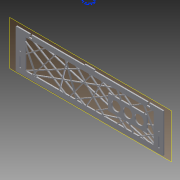
# Autodesk Inventor part: Panel_back
Saved by Autodesk Inventor 2013 (Build 170138000, 138)
## iProperties
Created: 2013-02-02
Part Number: Panel_back
Material: Aluminum 6061
Document SubType Name: Modeling
Designer: xylzlyx
Density: 1 g/cm^3
Author: xylzlyx
Autodesk Inventor part; units mm, degrees
ref_plane "YZ Plane" through (0, 0, 0) normal (1, 0, 0) x (0, 1, 0)
ref_plane "XZ Plane" through (0, 0, 0) normal (0, 1, 0) x (-1, 0, 0)
ref_plane "XY Plane" through (0, 0, 0) normal (0, 0, 1) x (1, 0, 0)
ref_plane "Work Plane1" through (-16.0071, 0, -12.7) normal (0, 0, 1) x (1, 0, 0)
sketch "Sketch1" plane through (-16.0071, 0, -12.7) normal (0, 0, 1) x (1, 0, 0)
  line L0 (0, -104.216) -> (0, -100.9921) construction
  line L1 (0, -100.9921) -> (381, -100.9921) construction
  line L2 (381, -100.9921) -> (381, -104.216) construction
  line L3 (381, -104.216) -> (0, -104.216) construction
  line L4 (381, 3.175) -> (381, 0) construction
  line L5 (381, 0) -> (0, 0) construction
  line L6 (0, 0) -> (0, 3.175) construction
  line L7 (0, 3.175) -> (381, 3.175) construction
  line L8 (381, -100.9921) -> (0, -100.9921)
  line L9 (0, -100.9921) -> (0, 0)
  line L10 (0, 0) -> (381, 0)
  line L11 (381, 0) -> (381, -100.9921)
  constraints: 24 end point, 5 horizontal, 4 coincident, 4 vertical, 2 parallel, 1 perpendicular, 7 other
extrude "BackPanel" add sketch "Sketch1" along normal blind 3.175
fillet "CornerFillet" radius 1 4 edges at (364.9929, -100.9921, -11.1125) (364.9929, 0, -11.1125) (-16.0071, 0, -11.1125) (-16.0071, -100.9921, -11.1125)
sketch "ScrewSlotSketch" plane through (-16.0071, 0, -9.525) normal (0, 0, 1) x (1, 0, 0)
  line L0 (0, -104.7759) -> (0, -101.5519) construction
  line L1 (0, -101.5519) -> (381, -101.5519) construction
  line L2 (381, -101.5519) -> (381, -104.7759) construction
  line L3 (381, -104.7759) -> (0, -104.7759) construction
  line L4 (381, 0) -> (0, 0) construction
  line L5 (0, 0) -> (0, 3.175) construction
  line L6 (0, 3.175) -> (381, 3.175) construction
  line L7 (381, 3.175) -> (381, 0) construction
  line L8 (341.0013, 3.175) -> (341.0013, -8.89)
  line L9 (341.0013, 3.175) -> (344.7986, 3.175)
  line L10 (344.7986, 3.175) -> (344.7986, -8.89)
  line L11 (344.7986, -8.89) -> (341.0013, -8.89)
  line L12 (342.9, -8.89) -> (342.9, 3.175) construction
  line L13 (346.9957, -8.89) -> (338.8042, -8.89)
  line L14 (338.8042, -8.89) -> (338.8042, -5.8579)
  line L15 (338.8042, -5.8579) -> (346.9957, -5.8579)
  line L16 (346.9957, -5.8579) -> (346.9957, -8.89)
  line L17 (36.2014, -8.89) -> (36.2014, 3.175)
  line L18 (36.2014, 3.175) -> (39.9987, 3.175)
  line L19 (39.9987, 3.175) -> (39.9987, -8.89)
  line L20 (39.9987, -8.89) -> (36.2014, -8.89)
  line L21 (42.1958, -8.89) -> (34.0043, -8.89)
  line L22 (42.1958, -8.89) -> (42.1958, -5.8579)
  line L23 (42.1958, -5.8579) -> (34.0043, -5.8579)
  line L24 (34.0043, -5.8579) -> (34.0043, -8.89)
  line L25 (368.3, -48.0974) -> (368.3, -1) projected
  line L26 (12.7, -1) -> (12.7, -48.0974) projected
  line L27 (368.3, -48.0974) -> (368.3, -1) projected
  point P0 (16.0071, 0)
  point P1 (38.1, 3.175)
  point P2 (38.1, -8.89)
  dimension "d3" = 12.065
  dimension "d5" = 3.7973
  dimension "d7" = 8.1915
  dimension "d8" = 3.0321
  dimension "d9" = 12.065
  dimension "d10" = 3.7973
  dimension "d12" = 8.1915
  dimension "d13" = 3.0321
  dimension "d22" = 25.4
  dimension "d23" = 25.4
  constraints: 50 end point, 13 parallel, 6 midpoint, 4 horizontal, 4 vertical, 3 collinear, 2 point on line, 1 perpendicular, 8 other
  measures "d3" distance of L8.start L8.end
  measures "d5" distance of L8.start L9.end
  measures "d7" distance of L13.start L13.end
  measures "d8" distance of L15.end L13.start
  measures "d9" distance of L17.start L17.end
  measures "d10" distance of L17.end L18.end
  measures "d12" distance of L21.start L21.end
  measures "d13" distance of L21.start L22.end
  measures "d22" distance between parallel lines of L12 L25
  measures "d23" distance from line of L26 point (38.1, 3.175)
extrude "ScrewSlotExtrusion" cut sketch "ScrewSlotSketch" against normal blind 3.175
fillet "SlotFillets" radius 0.5 16 edges at (328.7916, -5.8579, -11.1125) (328.7916, 0, -11.1125) (324.9943, 0, -11.1125) (324.9943, -5.8579, -11.1125) (330.9887, -5.8579, -11.1125) (322.7972, -5.8579, -11.1125) (330.9887, -8.89, -11.1125) (322.7972, -8.89, -11.1125) (20.1943, -5.8579, -11.1125) (17.9972, -5.8579, -11.1125) (20.1943, 0, -11.1125) (17.9972, -8.89, -11.1125) (23.9916, -5.8579, -11.1125) (23.9916, 0, -11.1125) (26.1887, -8.89, -11.1125) (26.1887, -5.8579, -11.1125)
sketch "ScrewHoleSketch" plane through (-16.0071, 0, -9.525) normal (0, 0, 1) x (1, 0, 0)
  line L0 (368.3, -48.5974) -> (371.475, -48.5974) projected
  line L1 (371.475, -52.3947) -> (368.3, -52.3947) projected
  line L2 (12.7, -52.3947) -> (9.525, -52.3947) projected
  line L3 (9.525, -48.5974) -> (12.7, -48.5974) projected
  line L4 (368.3, -48.5974) -> (368.3, -52.3947) construction
  line L5 (12.7, -48.5974) -> (12.7, -52.3947) construction
  line L6 (36.2014, -5.3579) -> (36.2014, -0.5) projected
  line L7 (344.7986, -0.5) -> (344.7986, -5.3579) projected
  point P0 (16.0071, 0)
  point P1 (369.8875, -50.496)
  point P2 (11.1125, -50.496)
  point P3 (368.3, -50.496)
  point P4 (369.8875, -48.5974)
  point P5 (11.1125, -48.5974)
  point P6 (12.7, -50.496)
  constraints: 4 end point, 4 midpoint, 3 parallel, 2 horizontal alignment, 2 vertical alignment
hole "Hole1" at (353.8804, -50.496, -9.525) at (-4.8946, -50.496, -9.525) direction (0, 0, -1) diameter 3.7973 end through all
sketch "BottomTabSketch" plane through (24.4916, 0, -12.7) normal (0, 1, 0) x (1, 0, 0)
  line L0 (137.3013, -3.175) -> (162.7013, -3.175)
  line L1 (162.7013, -3.175) -> (162.7013, 0)
  line L2 (162.7013, 0) -> (137.3013, 0)
  line L3 (137.3013, 0) -> (137.3013, -3.175)
  line L4 (137.5473, -3.429) -> (162.4553, -3.429) projected
  line L5 (137.0473, -0.246) -> (137.0473, -2.929) projected
  point P0 (0, 0)
  point P1 (-24.4916, -12.7)
  point P2 (150.0013, -3.175)
  point P3 (150.0013, -3.429)
  point P4 (137.3013, -1.5875)
  point P5 (137.0473, -1.5875)
  dimension "d32" = 25.4
  constraints: 8 end point, 4 midpoint, 2 horizontal alignment, 2 parallel, 1 horizontal, 1 perpendicular, 1 vertical alignment
  measures "d32" distance of L1.end L2.end
extrude "BottomTab" add sketch "BottomTabSketch" along normal blind 3.175
fillet "BottomTabFillet" radius 0.5 4 edges at (161.7929, 0, -11.1125) (161.7929, 3.175, -11.1125) (187.1929, 0, -11.1125) (187.1929, 3.175, -11.1125)
sketch "SlotSketch" plane through (-16.0071, 0, -9.525) normal (0, 0, 1) x (1, 0, 0)
  circle A0 centre (369.8875, -50.496) radius 1.8986 projected
  circle A1 centre (11.1125, -50.496) radius 1.8986 projected
  line L0 (0, -104.7759) -> (0, -101.5519) construction
  line L1 (0, -101.5519) -> (381, -101.5519) construction
  line L2 (381, -101.5519) -> (381, -104.7759) construction
  line L3 (381, -104.7759) -> (0, -104.7759) construction
  line L4 (371.729, -88.6981) -> (368.046, -88.6981)
  line L5 (368.046, -88.6981) -> (368.046, -62.7901)
  line L6 (368.046, -62.7901) -> (371.729, -62.7901)
  line L7 (371.729, -62.7901) -> (371.729, -88.6981)
  line L8 (12.954, -88.6981) -> (9.271, -88.6981)
  line L9 (9.271, -88.6981) -> (9.271, -62.7901)
  line L10 (9.271, -62.7901) -> (12.954, -62.7901)
  line L11 (12.954, -62.7901) -> (12.954, -88.6981)
  line L12 (1, -100.9921) -> (380, -100.9921) projected
  line L13 (203.2, 0.5) -> (203.2, 2.675) projected
  line L14 (11.1125, -50.496) -> (11.1125, -100.9921) construction
  line L15 (369.8875, -50.496) -> (369.8875, -100.9921) construction
  point P0 (16.0071, 0)
  point P1 (11.1125, -75.7441)
  point P2 (12.954, -75.7441)
  point P3 (11.1125, -62.7901)
  point P4 (369.8875, -75.7441)
  point P5 (371.729, -75.7441)
  point P6 (369.8875, -62.7901)
  dimension "d37" = 25.908
  dimension "d39" = 3.683
  dimension "d40" = 25.908
  dimension "d41" = 3.683
  constraints: 28 end point, 6 midpoint, 6 parallel, 4 horizontal, 2 horizontal alignment, 2 perpendicular, 2 point on line, 2 vertical, 2 vertical alignment, 4 other
  measures "d37" distance of L4.end L5.end
  measures "d39" distance of L4.start L4.end
  measures "d40" distance of L10.end L8.start
  measures "d41" distance of L8.start L8.end
extrude "Slots" cut sketch "SlotSketch" against normal blind 3.175 contours L4 L5 L6 L7 | L8 L9 L10 L11
fillet "Fillet4" radius 0.5 8 edges at (355.7219, -88.6981, -11.1125) (352.0389, -88.6981, -11.1125) (352.0389, -62.7901, -11.1125) (355.7219, -62.7901, -11.1125) (-6.7361, -62.7901, -11.1125) (-3.0531, -62.7901, -11.1125) (-6.7361, -88.6981, -11.1125) (-3.0531, -88.6981, -11.1125)
sketch "Sketch6" plane through (-16.0071, 0, -9.525) normal (0, 0, 1) x (1, 0, 0)
  line L0 (1, -100.9921) -> (380, -100.9921) projected
  line L1 (380, 0) -> (345.2986, 0) projected
  circle A0 centre (369.8875, -50.496) radius 1.8986 projected
  circle A1 centre (11.1125, -50.496) radius 1.8986 projected
  line L2 (357.1875, -88.2921) -> (23.8125, -88.2921)
  line L3 (23.8125, -88.2921) -> (23.8125, -12.7)
  line L4 (23.8125, -12.7) -> (357.1875, -12.7)
  line L5 (357.1875, -12.7) -> (357.1875, -88.2921)
  point P0 (16.0071, 0)
  dimension "d45" = 12.7
  dimension "d46" = 12.7
  dimension "d47" = 12.7
  dimension "d48" = 12.7
  constraints: 8 end point, 2 parallel, 1 horizontal, 1 perpendicular
  measures "d45" distance from line of L0 L2.start
  measures "d46" distance from line of L1 L4.end
  measures "d47" distance from line of A0.centre L5
  measures "d48" horizontal distance of A1.centre L3.end
extrude "InsideGap" cut sketch "Sketch6" against normal blind 25.4 contours L2 L3 L4 L5
fillet "InsideGapFillet" radius 0.5 4 edges at (341.1804, -88.2921, -11.1125) (341.1804, -12.7, -11.1125) (7.8054, -12.7, -11.1125) (7.8054, -88.2921, -11.1125)
sketch "Sketch7" plane through (-16.0071, 0, -9.525) normal (0, 0, 1) x (1, 0, 0)
  line L0 (357.1875, -13.2) -> (357.1875, -87.7921) projected
  line L1 (356.6875, -88.2921) -> (24.3125, -88.2921) projected
  line L2 (23.8125, -87.7921) -> (23.8125, -13.2) projected
  line L3 (24.3125, -12.7) -> (356.6875, -12.7) projected
  line L4 (340.5013, 0) -> (203.7, 0) projected
  line L5 (354.4479, -12.7) -> (264.3608, -88.2921)
  line L6 (327.4775, -12.7) -> (206.5049, -88.2921)
  line L7 (285.5675, -12.7) -> (154.6382, -88.2921)
  line L8 (254.9043, -12.7) -> (47.2168, -88.2921)
  line L9 (225.9343, -12.7) -> (182.8154, -88.2921)
  line L10 (169.3262, -12.7) -> (27.1582, -88.2921)
  line L11 (132.4925, -12.7) -> (113.0758, -88.2921)
  line L12 (77.2875, -12.7) -> (23.8125, -52.9963)
  line L13 (357.1875, -66.5903) -> (320.5833, -88.2921)
  line L14 (357.1875, -66.5903) -> (357.1875, -64.228)
  line L15 (357.1875, -64.228) -> (316.5989, -88.2921)
  line L16 (316.5989, -88.2921) -> (320.5833, -88.2921)
  line L17 (351.2867, -12.7) -> (261.1996, -88.2921)
  line L18 (261.1996, -88.2921) -> (264.3608, -88.2921)
  line L19 (354.4479, -12.7) -> (351.2867, -12.7)
  line L20 (327.4775, -12.7) -> (323.643, -12.7)
  line L21 (323.643, -12.7) -> (202.6704, -88.2921)
  line L22 (202.6704, -88.2921) -> (206.5049, -88.2921)
  line L23 (285.5675, -12.7) -> (281.5035, -12.7)
  line L24 (281.5035, -12.7) -> (150.5742, -88.2921)
  line L25 (150.5742, -88.2921) -> (154.6382, -88.2921)
  line L26 (254.9043, -12.7) -> (248.9631, -12.7)
  line L27 (248.9631, -12.7) -> (41.2756, -88.2921)
  line L28 (41.2756, -88.2921) -> (47.2168, -88.2921)
  line L29 (225.9343, -12.7) -> (223.595, -12.7)
  line L30 (223.595, -12.7) -> (180.476, -88.2921)
  line L31 (180.476, -88.2921) -> (182.8154, -88.2921)
  line L32 (169.3262, -12.7) -> (164.998, -12.7)
  line L33 (164.998, -12.7) -> (22.83, -88.2921)
  line L34 (22.83, -88.2921) -> (27.1582, -88.2921)
  line L35 (132.4925, -12.7) -> (130.3945, -12.7)
  line L36 (130.3945, -12.7) -> (110.9779, -88.2921)
  line L37 (110.9779, -88.2921) -> (113.0758, -88.2921)
  line L38 (77.2875, -12.7) -> (73.911, -12.7)
  line L39 (73.911, -12.7) -> (23.8125, -50.452)
  line L40 (23.8125, -50.452) -> (23.8125, -52.9963)
  line L41 (195.7846, -12.7) -> (140.0963, -88.2921)
  line L42 (140.0963, -88.2921) -> (137.5725, -88.2921)
  line L43 (137.5725, -88.2921) -> (193.2608, -12.7)
  line L44 (193.2608, -12.7) -> (195.7846, -12.7)
  line L45 (103.9917, -12.7) -> (43.8325, -88.2921)
  line L46 (43.8325, -88.2921) -> (41.2356, -88.2921)
  line L47 (41.2356, -88.2921) -> (101.3947, -12.7)
  line L48 (101.3947, -12.7) -> (103.9917, -12.7)
  arc A0 (357.1875, -13.2) -> (356.6875, -12.7) centre (356.6875, -13.2) ccw projected
  line L49 (357.1875, -46.5241) -> (225.1649, -88.2921)
  line L50 (357.1875, -46.5241) -> (357.1875, -44.3928)
  line L51 (357.1875, -44.3928) -> (218.4282, -88.2921)
  line L52 (218.4282, -88.2921) -> (225.1649, -88.2921)
  point P0 (16.0071, 0)
  dimension "d52" = 2.2396
  dimension "d53" = 29.21
  dimension "d54" = 71.12
  dimension "d55" = 101.7832
  dimension "d56" = 130.7532
  dimension "d57" = 187.3613
  dimension "d58" = 224.195
  dimension "d59" = 279.4
  dimension "d60" = 53.3903
  dimension "d61" = 59.337
  dimension "d62" = 140
  dimension "d63" = 148
  dimension "d64" = 150
  dimension "d65" = 160
  dimension "d66" = 119.701
  dimension "d67" = 152
  dimension "d68" = 104.406
  dimension "d69" = 143
  dimension "d70" = 2.032
  dimension "d71" = 2.032
  dimension "d72" = 2.032
  dimension "d73" = 2.032
  dimension "d74" = 2.032
  dimension "d75" = 2.032
  dimension "d76" = 2.032
  dimension "d77" = 2.032
  dimension "d78" = 2.032
  dimension "d79" = 2.032
  dimension "d80" = 160.9029
  dimension "d81" = 126.379
  dimension "d82" = 252.6958
  dimension "d83" = 128.514
  dimension "d84" = 2.032
  dimension "d122" = 33.324
  dimension "d123" = 72.444
  dimension "d124" = 2.032
  constraints: 96 end point, 17 parallel, 14 horizontal, 3 collinear, 3 point on line, 27 other
  measures "d52" distance of L5.start A0.end
  measures "d53" distance of L6.start A0.end
  measures "d54" distance of L7.start A0.end
  measures "d55" distance of L8.start A0.end
  measures "d56" distance of L9.start A0.end
  measures "d57" distance of L10.start A0.end
  measures "d58" distance of L11.start A0.end
  measures "d59" distance of L12.start A0.end
  measures "d60" distance of L0.start L13.start
  measures "d61" angle of L0 L13
  measures "d62" angle to the sketch x axis of L5
  measures "d63" angle to the sketch x axis of L6
  measures "d64" angle to the sketch x axis of L7
  measures "d65" angle to the sketch x axis of L8
  measures "d66" angle to the sketch x axis of L9
  measures "d67" angle to the sketch x axis of L10
  measures "d68" angle to the sketch x axis of L11
  measures "d69" angle to the sketch x axis of L12
  measures "d70" distance between parallel lines of L15 L13
  measures "d71" distance between parallel lines of L5 L17
  measures "d72" distance between parallel lines of L6 L21
  measures "d73" distance between parallel lines of L7 L24
  measures "d74" distance between parallel lines of L8 L27
  measures "d75" distance between parallel lines of L9 L30
  measures "d76" distance between parallel lines of L10 L33
  measures "d77" distance between parallel lines of L11 L36
  measures "d78" distance between parallel lines of L12 L39
  measures "d79" distance between parallel lines of L41 L43
  measures "d80" distance of A0.end L41.start
  measures "d81" angle to the sketch x axis of L41
  measures "d82" distance of A0.end L45.start
  measures "d83" angle to the sketch x axis of L45
  measures "d84" distance between parallel lines of L45 L47
  measures "d122" vertical distance of A0.centre L49.start
  measures "d123" angle of L0 L49
  measures "d124" distance between parallel lines of L49 L51
extrude "Hash1" add sketch "Sketch7" against normal blind 3.175 contours L0 L49 L5 L51 | L51 L17 L3 L5 | L5 L49 L17 L51 | L0 L13 L1 L15 | L5 L1 L17 L49 | L17 L49 L1 L51 | L6 L1 L21 L3 | L7 L9 L24 L3 | L1 L30 L7 L9 | L7 L30 L24 L9 | L8 L9 L27 L3 | L24 L30 L8 L9 | L7 L1 L24 L30 | L8 L30 L27 L9 | L9 L27 L30 L3 | L8 L41 L27 L30 | L1 L43 L8 L41 | L8 L43 L27 L41 | L41 L27 L43 L3 | L8 L11 L27 L43 | L1 L36 L8 L11 | L8 L36 L27 L11 | L10 L11 L33 L3 | L27 L36 L10 L11 | L8 L1 L45 L27 L36 | L10 L36 L33 L11 | L1 L27 L45 | L11 L33 L36 L3 | L10 L45 L33 L36 | L27 L1 L47 L10 L45 | L10 L47 L33 L45 | L45 L33 L47 L3 | L10 L1 L34 L33 L47 | L12 L2 L39 L3
sketch "Sketch8" plane through (-16.0071, 0, -9.525) normal (0, 0, 1) x (1, 0, 0)
  line L0 (77.2875, -12.7) -> (101.3947, -12.7) projected
  line L1 (169.3262, -12.7) -> (193.2608, -12.7) projected
  line L2 (137.5725, -88.2921) -> (113.0758, -88.2921) projected
  line L3 (110.9779, -88.2921) -> (320.5833, -88.2921) projected
  line L4 (356.6875, -88.2921) -> (140.0963, -88.2921) projected
  line L5 (357.1875, -66.5903) -> (357.1875, -87.7921) projected
  line L6 (316.5989, -88.2921) -> (206.5049, -88.2921) projected
  line L7 (261.1996, -88.2921) -> (154.6382, -88.2921) projected
  line L8 (285.5675, -12.7) -> (323.643, -12.7) projected
  line L9 (254.9043, -12.7) -> (281.5035, -12.7) projected
  line L10 (150.5742, -88.2921) -> (182.8154, -88.2921) projected
  line L11 (132.4925, -12.7) -> (164.998, -12.7) projected
  line L12 (225.9343, -12.7) -> (248.9631, -12.7) projected
  line L13 (23.8125, -50.452) -> (23.8125, -13.2) projected
  line L14 (24.3125, -12.7) -> (73.911, -12.7) projected
  line L15 (327.4775, -12.7) -> (351.2867, -12.7) projected
  line L16 (340.5013, 0) -> (203.7, 0) projected
  line L17 (23.8125, -34.0474) -> (50.1687, -88.2921)
  line L18 (23.8125, -24.8637) -> (123.9909, -88.2921)
  line L19 (42.1433, -12.7) -> (173.0726, -88.2921)
  line L20 (76.4841, -12.7) -> (332.9933, -88.2921)
  line L21 (126.5475, -12.7) -> (155.5646, -88.2921)
  line L22 (153.8525, -12.7) -> (225.0869, -88.2921)
  line L23 (187.5335, -12.7) -> (281.551, -88.2921)
  line L24 (218.779, -12.7) -> (357.1875, -88.2921)
  line L25 (259.8239, -12.7) -> (300.7816, -88.2921)
  line L26 (273.2325, -12.7) -> (357.1875, -77.3074)
  line L27 (357.1875, -61.6757) -> (328.9114, -12.7)
  line L28 (357.1875, -61.6757) -> (357.1875, -57.6117)
  line L29 (357.1875, -57.6117) -> (331.2577, -12.7)
  line L30 (331.2577, -12.7) -> (328.9114, -12.7)
  line L31 (300.7816, -88.2921) -> (303.0927, -88.2921)
  line L32 (303.0927, -88.2921) -> (262.135, -12.7)
  line L33 (262.135, -12.7) -> (259.8239, -12.7)
  line L34 (281.551, -88.2921) -> (284.7939, -88.2921)
  line L35 (284.7939, -88.2921) -> (190.7764, -12.7)
  line L36 (190.7764, -12.7) -> (187.5335, -12.7)
  line L37 (225.0869, -88.2921) -> (227.8789, -88.2921)
  line L38 (227.8789, -88.2921) -> (156.6446, -12.7)
  line L39 (156.6446, -12.7) -> (153.8525, -12.7)
  line L40 (155.5646, -88.2921) -> (157.7411, -88.2921)
  line L41 (157.7411, -88.2921) -> (128.7241, -12.7)
  line L42 (128.7241, -12.7) -> (126.5475, -12.7)
  line L43 (332.9933, -88.2921) -> (340.1817, -88.2921)
  line L44 (340.1817, -88.2921) -> (83.6725, -12.7)
  line L45 (83.6725, -12.7) -> (76.4841, -12.7)
  line L46 (123.9909, -88.2921) -> (127.7895, -88.2921)
  line L47 (127.7895, -88.2921) -> (23.8125, -22.4586)
  line L48 (23.8125, -22.4586) -> (23.8125, -24.8637)
  line L49 (173.0726, -88.2921) -> (177.1366, -88.2921)
  line L50 (177.1366, -88.2921) -> (46.2073, -12.7)
  line L51 (46.2073, -12.7) -> (42.1433, -12.7)
  line L52 (50.1687, -88.2921) -> (52.4278, -88.2921)
  line L53 (52.4278, -88.2921) -> (23.8125, -29.3978)
  line L54 (23.8125, -29.3978) -> (23.8125, -34.0474)
  line L55 (195.7846, -12.7) -> (223.595, -12.7) projected
  line L56 (357.1875, -77.3074) -> (357.1875, -74.7434)
  line L57 (357.1875, -74.7434) -> (276.5644, -12.7)
  line L58 (276.5644, -12.7) -> (273.2325, -12.7)
  line L59 (357.1875, -88.2921) -> (357.1875, -85.9768)
  line L60 (357.1875, -85.9768) -> (223.0183, -12.7)
  line L61 (223.0183, -12.7) -> (218.779, -12.7)
  point P0 (43.8325, -88.2921)
  point P1 (158.6823, -88.2921)
  point P2 (16.0071, 0)
  dimension "d87" = 20.8474
  dimension "d88" = 11.6637
  dimension "d89" = 154.086
  dimension "d90" = 122.34
  dimension "d91" = 17.8308
  dimension "d92" = 52.1716
  dimension "d93" = 150
  dimension "d94" = 163.58
  dimension "d95" = 102.235
  dimension "d96" = 111
  dimension "d97" = 129.54
  dimension "d98" = 133.3
  dimension "d99" = 163.221
  dimension "d100" = 141.2
  dimension "d101" = 194.4665
  dimension "d103" = 235.5114
  dimension "d104" = 118.45
  dimension "d105" = 248.92
  dimension "d106" = 142.42
  dimension "d107" = 304.5989
  dimension "d108" = 120
  dimension "d109" = 2.032
  dimension "d111" = 2.032
  dimension "d112" = 2.032
  dimension "d114" = 2.032
  dimension "d115" = 2.032
  dimension "d116" = 2.032
  dimension "d117" = 2.032
  dimension "d118" = 2.032
  dimension "d119" = 2.032
  dimension "d125" = 2.032
  dimension "d126" = 2.032
  constraints: 88 end point, 23 point on line, 20 collinear, 13 parallel
  measures "d87" distance of L13.end L17.start
  measures "d88" distance of L13.end L18.start
  measures "d89" angle of L13 L17
  measures "d90" angle of L13 L18
  measures "d91" distance of L14.start L19.start
  measures "d92" distance of L14.start L20.start
  measures "d93" angle of L14 L19
  measures "d94" angle of L0 L20
  measures "d95" distance of L14.start L21.start
  measures "d96" angle of L11 L21
  measures "d97" distance of L14.start L22.start
  measures "d98" angle of L11 L22
  measures "d99" distance of L14.start L23.start
  measures "d100" angle of L1 L23
  measures "d101" distance of L14.start L24.start
  measures "d103" distance of L14.start L25.start
  measures "d104" angle of L12 L25
  measures "d105" distance of L14.start L26.start
  measures "d106" angle of L8 L26
  measures "d107" distance of L14.start L27.end
  measures "d108" angle of L15 L27
  measures "d109" distance between parallel lines of L27 L29
  measures "d111" distance between parallel lines of L25 L32
  measures "d112" distance between parallel lines of L23 L35
  measures "d114" distance between parallel lines of L22 L38
  measures "d115" distance between parallel lines of L21 L41
  measures "d116" distance between parallel lines of L20 L44
  measures "d117" distance between parallel lines of L18 L47
  measures "d118" distance between parallel lines of L19 L50
  measures "d119" distance between parallel lines of L17 L53
  measures "d125" distance between parallel lines of L26 L57
  measures "d126" distance between parallel lines of L24 L60
extrude "Hash2" add sketch "Sketch8" against normal blind 3.175 contours L0 L44 L21 L20 L45 | L44 L41 L20 L21 | L21 L42 L41 L44 | L20 L41 L50 L21 | L44 L22 L20 L41 | L50 L41 L19 L21 | L21 L19 L14 L50 | L44 L38 L20 L22 | L22 L11 L38 L44 | L20 L38 L3 L22 | L50 L3 L19 L41 | L19 L41 L3 L21 | L44 L23 L20 L38 | L44 L35 L20 L23 | L23 L1 L35 L44 | L20 L35 L3 L23 | L44 L25 L20 L35 | L44 L32 L20 L25 | L25 L24 L32 L44 | L20 L32 L3 L25 | L25 L60 L32 L24 | L24 L55 L60 L25 | L44 L4 L20 L32 | L32 L60 L5 L59 L24 | L25 L9 L32 L60 | L9 L57 L5 L26 | L2 L18 L13 L47 | L13 L53 L52 L17 | L15 L29 L28 L27
sketch "Sketch9" plane through (-16.0071, 0, -9.525) normal (0, 0, 1) x (1, 0, 0)
  circle A0 centre (369.8875, -50.496) radius 1.8986 projected
  line L0 (1, -100.9921) -> (380, -100.9921) projected
  line L1 (381, -99.9921) -> (381, -1) projected
  line L2 (380, 0) -> (345.2986, 0) projected
  line L3 (339.0875, -70.496) -> (239.0875, -70.496)
  line L4 (239.0875, -70.496) -> (239.0875, -30.496)
  line L5 (239.0875, -30.496) -> (339.0875, -30.496)
  line L6 (339.0875, -30.496) -> (339.0875, -70.496)
  point P0 (16.0071, 0)
  point P1 (289.0875, -50.496)
  point P2 (259.0875, -50.496)
  point P3 (319.0875, -50.496)
  point P4 (339.0875, -50.496)
  point P5 (289.0875, -70.496)
  dimension "d127" = 30
  dimension "d129" = 30
  dimension "d130" = 50.8
  dimension "d131" = 20
  dimension "d132" = 20
  constraints: 8 end point, 4 horizontal alignment, 4 parallel, 2 midpoint, 1 vertical alignment
  measures "d127" distance of point (289.087, -50.496) point (319.087, -50.496)
  measures "d129" distance of point (289.087, -50.496) point (259.087, -50.496)
  measures "d130" distance of point (319.087, -50.496) A0.centre
  measures "d131" distance from line of L6 point (319.087, -50.496)
  measures "d132" distance from line of L3 point (319.087, -50.496)
extrude "BackButtonMount" add sketch "Sketch9" against normal blind 3.175 contours L3 L4 L5 L6
sketch "Sketch10" plane through (-16.0071, 0, -9.525) normal (0, 0, 1) x (1, 0, 0)
  circle A0 centre (369.8875, -50.496) radius 1.8986 projected
  point P0 (16.0071, 0)
  point P1 (319.0875, -50.496)
  point P2 (289.0875, -50.496)
  point P3 (259.0875, -50.496)
  point P4 (289.0875, -50.496)
  dimension "d135" = 30
  dimension "d137" = 30
  constraints: 3 horizontal alignment, 1 coincident
  measures "d135" distance of point (319.087, -50.496) point (289.087, -50.496)
  measures "d137" distance of point (259.087, -50.496) point (289.087, -50.496)
hole "BackButtonHoles" at (303.0804, -50.496, -9.525) at (273.0804, -50.496, -9.525) at (243.0804, -50.496, -9.525) direction (0, 0, -1) diameter 24 end through all
equation "\"d3\" = ScrewLen"
equation "\"d5\" = ScrewHoleD"
equation "\"d7\" = NutFlatsGap"
equation "\"d8\" = NutHeightGap"
equation "\"d9\" = ScrewLen"
equation "\"d10\" = ScrewHoleD"
equation "\"d12\" = NutFlatsGap"
equation "\"d13\" = NutHeightGap"
equation "\"d22\" = ScrewHoleDist"
equation "\"d23\" = ScrewHoleDist"
equation "\"d24\" = SlotFilletRad"
equation "\"d25\" = ScrewHoleD"
equation "\"d32\" = TabLength"
equation "\"d36\" = SlotFilletRad"
equation "\"d37\" = SlotLength"
equation "\"d39\" = SlotWidth"
equation "\"d40\" = SlotLength"
equation "\"d41\" = SlotWidth"
equation "\"d44\" = SlotFilletRad"
equation "\"d45\" = EdgeThickness"
equation "\"d46\" = EdgeThickness"
equation "\"d47\" = EdgeThickness"
equation "\"d48\" = EdgeThickness"
equation "\"d51\" = SlotFilletRad"
equation "\"ScrewLen\" = 12.065"
equation "\"ScrewHoleD\" = 3.7973"
equation "\"NutFlatsGap\" = 8.1915"
equation "\"NutHeightGap\" = 3.032125"
equation "\"ScrewHoleDist\" = 25.4"
equation "\"SlotFilletRad\" = 0.5"
equation "\"TabLength\" = 25.4"
equation "\"SlotLength\" = 25.908"
equation "\"SlotWidth\" = 3.683"
equation "\"EdgeThickness\" = 12.7"
body "Solid1"
